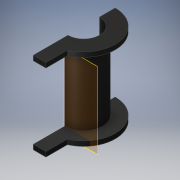
# Autodesk Inventor part: Test2
Saved by Autodesk Inventor 2019 (Build 230136000, 136)
## iProperties
Created: 2020-04-08
Part Number: Test2
Material: ABS Plastic
Document SubType Name: Modeling
Designer: Erle
Density: 1.06 g/cm^3
Appearance: Glossy - Black
Mass: 1.1218 g
Surface Area: 14.6771 cm^2
Volume: 1.05831 cm^3
Author: Erle
Autodesk Inventor part; units mm, degrees
ref_plane "YZ Plane" through (0, 0, 0) normal (1, 0, 0) x (0, 1, 0)
ref_plane "XZ Plane" through (0, 0, 0) normal (0, 1, 0) x (-1, 0, 0)
sketch "Sketch1" plane through (0, 0, 0) normal (0, 1, 0) x (-1, 0, 0)
  circle A0 centre (0, 0) radius 10
  dimension "d0" = 20
  constraints: 1 centre point, 1 coincident
  measures "d0" diameter of A0
extrude "Extrusion1" add sketch "Sketch1" along normal blind 26
sketch "Sketch2" plane through (0, 0, 0) normal (0, -1, 0) x (1, 0, 0)
  point P0 (0, 0)
  point P1 (0, 0)
  constraints: 1 coincident
hole "Hole1" at (0, 0, 0) direction (0, 1, 0) diameter 5.5 end through all counterbore diameter 10 counterbore depth 5.5 clearance for "Socket Head Cap Screw DIN EN ISO 4762" size "M5" standard "DIN"
sketch "Sketch3" plane through (0, 0, 0) normal (1, 0, 0) x (0, 1, 0)
  line L0 (24.5, 10) -> (1.5, 10)
  line L1 (1.5, 10) -> (1.5, 6)
  line L2 (1.5, 6) -> (24.5, 6)
  line L3 (24.5, 6) -> (24.5, 10)
  line L4 (26, -10) -> (26, 10) projected
  line L5 (-4.4, 0) -> (26.4, 0) projected
  point P0 (0, 0)
  dimension "d10" = 6
  dimension "d11" = 1.5
  dimension "d12" = 1.5
  constraints: 8 end point, 2 parallel, 1 horizontal, 1 horizontal alignment, 1 perpendicular
  measures "d10" vertical distance of point (0, 0) L1.end
  measures "d11" distance from line of point (0, 0) L1
  measures "d12" distance between parallel lines of L4 L3
revolve "Revolution1" cut sketch "Sketch3" angle 360 about axis through (0, -10, 0) along (0, 1, 0)
sketch "Sketch5" plane through (0, 26, 0) normal (0, 1, 0) x (1, 0, 0)
  circle A0 centre (0, 0) radius 2.75 projected
  constraints: 1 coincident
hole "Hole2" at (0, 26, 0) direction (0, -1, 0) diameter 5.5 end through all counterbore diameter 10 counterbore depth 5.5 clearance for "Socket Head Cap Screw DIN EN ISO 4762" size "M5" standard "DIN"
sketch "Sketch7" plane through (0, 0, 0) normal (1, 0, 0) x (0, 1, 0)
  line L0 (-12.4894, -25.9847) -> (40.6535, -25.9847)
  line L1 (40.6535, -25.9847) -> (40.6535, 26.2362)
  line L2 (40.6535, 26.2362) -> (-12.4894, 26.2362)
  line L3 (-12.4894, 26.2362) -> (-12.4894, -25.9847)
  point P0 (0, 0)
  constraints: 8 end point, 2 parallel, 1 horizontal, 1 perpendicular
extrude "Extrusion3" cut sketch "Sketch7" against normal blind 15
ref_plane "Work Plane1" through (0, 0, 6) normal (0, 0, 1) x (1, 0, 0)
sketch "Sketch8" plane through (0, 0, 6) normal (0, 0, 1) x (1, 0, 0)
  line L0 (0, 0) -> (10, 0) projected
  line L1 (0, 1.5) -> (10, 1.5) projected
  line L2 (0, 0) -> (4, 0)
  line L3 (4, 0) -> (4, 1.5)
  line L4 (4, 1.5) -> (0, 1.5)
  line L5 (0, 1.5) -> (0, 0)
  line L6 (0, 20.5) -> (0, 26) projected
  line L7 (10, 24.5) -> (0, 24.5) projected
  line L8 (0, 26) -> (4, 26)
  line L9 (4, 26) -> (4, 24.5)
  line L10 (4, 24.5) -> (0, 24.5)
  line L11 (0, 24.5) -> (0, 26)
  dimension "d26" = 4
  constraints: 16 end point, 4 parallel, 2 horizontal, 2 perpendicular, 2 point on line, 1 vertical alignment
  measures "d26" distance of L6.end L8.end
extrude "Extrusion4" add sketch "Sketch8" along normal blind 10
body "Solid1"
